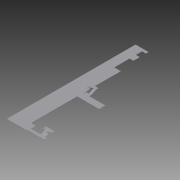
# Autodesk Inventor part: LabVIEWM0.5
Saved by Autodesk Inventor 2013 SP2 (Build 170200200, 200)
## iProperties
Created: 2014-11-17
Part Number: LabVIEWM0.5
Material: 常规
Document SubType Name: Modeling
Designer: 振胜
Density: 1 g/cm^3
Author: 振胜
Autodesk Inventor part; units mm, degrees
ref_plane "工作平面1" through (0, 0, 0) normal (0, 0, 1) x (1, 0, 0)
sketch "草图1" plane through (0, 0, 0) normal (0, 0, 1) x (1, 0, 0)
  line L0 (0, 0) -> (60, 0)
  line L1 (60, 0) -> (60, -1169.8)
  line L2 (60, -1169.8) -> (0, -1169.8)
  line L3 (0, -1169.8) -> (0, 0)
  line L4 (0, -80.6) -> (60, -80.6)
  line L5 (0, -191.9) -> (60, -191.9)
  line L6 (0, -276.5) -> (60, -276.5)
  line L7 (0, -335.9) -> (60, -335.9)
  line L8 (0, -420.6) -> (60, -420.6)
  line L9 (0, -550.6) -> (60, -550.6)
  line L10 (0, -677.8) -> (60, -677.8)
  line L11 (0, -782.9) -> (60, -782.9)
  line L12 (0, -839.5) -> (60, -839.5)
  line L13 (0, -923.6) -> (60, -923.6)
  line L14 (0, -1007.7) -> (60, -1007.7)
  line L15 (0, -1091.2) -> (60, -1091.2)
  line L16 (60, 0) -> (118.4, 0)
  line L17 (118.4, 0) -> (118.4, -23.7)
  line L18 (118.4, -23.7) -> (83.4, -23.7)
  line L19 (83.4, -23.7) -> (83.4, -79.7)
  line L20 (83.4, -79.7) -> (118.4, -79.7)
  line L21 (118.4, -79.7) -> (118.4, -137.6)
  line L22 (118.4, -137.6) -> (83.4, -137.6)
  line L23 (83.4, -137.6) -> (83.4, -276.5)
  line L24 (83.4, -276.5) -> (142.9, -276.5)
  line L25 (142.9, -276.5) -> (142.9, -379.5)
  line L26 (83.4, -276.5) -> (83.4, -379.5)
  line L27 (83.4, -379.5) -> (142.9, -379.5)
  line L28 (142.9, -379.5) -> (142.9, -463)
  line L29 (142.9, -463) -> (83.4, -463)
  line L30 (83.4, -463) -> (83.4, -379.5)
  line L31 (142.9, -463) -> (142.9, -566.2)
  line L32 (142.9, -566.2) -> (83.4, -566.2)
  line L33 (83.4, -566.2) -> (83.4, -463)
  line L34 (142.9, -566.2) -> (146.7, -566.2)
  line L35 (146.7, -566.2) -> (146.7, -616.2)
  line L36 (146.7, -616.2) -> (192.5, -616.2)
  line L37 (192.5, -616.2) -> (192.5, -673.2)
  line L38 (192.5, -616.2) -> (342.5, -616.2)
  line L39 (342.5, -616.2) -> (342.5, -673.2)
  line L40 (342.5, -673.2) -> (143.4, -673.2)
  line L41 (143.4, -673.2) -> (83.4, -673.2)
  line L42 (83.4, -673.2) -> (83.4, -1092.3)
  line L43 (83.4, -1092.3) -> (143.4, -1092.3)
  line L44 (143.4, -1092.3) -> (143.4, -673.2)
  line L45 (83.4, -754.3) -> (143.4, -754.3)
  line L46 (143.4, -837.8) -> (83.4, -837.8)
  line L47 (83.4, -893.6) -> (143.4, -893.6)
  line L48 (143.4, -978.3) -> (83.4, -978.3)
  line L49 (60, -1169.8) -> (188.1, -1169.8)
  line L50 (188.1, -1169.8) -> (188.1, -1092.3)
  line L51 (188.1, -1092.3) -> (143.4, -1092.3)
  line L52 (83.4, -1092.3) -> (83.4, -1117.3)
  line L53 (83.4, -1117.3) -> (188.1, -1117.3)
  line L54 (98.6, -1092.3) -> (98.6, -1117.3)
  line L55 (114.5, -1092.3) -> (114.5, -1117.3)
  line L56 (143.4, -1092.3) -> (143.4, -1117.3)
  line L57 (166.2, -1092.3) -> (166.2, -1117.3)
  line L58 (188.1, -1163.6) -> (336, -1163.6)
  line L59 (188.1, -1137.1) -> (336, -1137.1)
  line L60 (336, -1137.1) -> (336, -1163.6)
  dimension "d1" = 60
  dimension "d2" = 80.6
  dimension "d3" = 111.3
  dimension "d4" = 84.6
  dimension "d5" = 59.4
  dimension "d6" = 84.7
  dimension "d7" = 130
  dimension "d8" = 127.2
  dimension "d9" = 105.1
  dimension "d10" = 56.6
  dimension "d11" = 84.1
  dimension "d12" = 84.1
  dimension "d13" = 83.5
  dimension "d14" = 78.6
  dimension "d15" = 58.4
  dimension "d16" = 23.7
  dimension "d17" = 35
  dimension "d18" = 56
  dimension "d19" = 57.9
  dimension "d20" = 35
  dimension "d21" = 138.9
  dimension "d22" = 59.5
  dimension "d23" = 103
  dimension "d24" = 83.5
  dimension "d25" = 103.2
  dimension "d26" = 59.5
  dimension "d27" = 3.8
  dimension "d28" = 50
  dimension "d29" = 45.8
  dimension "d30" = 57
  dimension "d31" = 150
  dimension "d32" = 57
  dimension "d33" = 199.1
  dimension "d34" = 60
  dimension "d36" = 81.1
  dimension "d37" = 83.5
  dimension "d38" = 55.8
  dimension "d39" = 84.7
  dimension "d40" = 114
  dimension "d41" = 128.1
  dimension "d42" = 25
  dimension "d43" = 15.2
  dimension "d44" = 15.9
  dimension "d45" = 28.9
  dimension "d46" = 22.8
  dimension "d47" = 21.9
  dimension "d48" = 147.9
  dimension "d49" = 6.2
  dimension "d50" = 26.5
  constraints: 118 end point, 34 perpendicular, 19 point on line, 14 parallel, 13 horizontal, 30 other
  measures "d1" distance of L0.start L0.end
  measures "d2" distance between parallel lines of L4 L0
  measures "d3" distance between parallel lines of L5 L4
  measures "d4" distance between parallel lines of L6 L5
  measures "d5" distance between parallel lines of L7 L6
  measures "d6" distance between parallel lines of L8 L7
  measures "d7" distance between parallel lines of L9 L8
  measures "d8" distance between parallel lines of L10 L9
  measures "d9" distance between parallel lines of L11 L10
  measures "d10" distance between parallel lines of L12 L11
  measures "d11" distance between parallel lines of L13 L12
  measures "d12" distance between parallel lines of L14 L13
  measures "d13" distance between parallel lines of L15 L14
  measures "d14" distance between parallel lines of L2 L15
  measures "d15" distance of L0.end L16.end
  measures "d16" distance of L16.end L17.end
  measures "d17" distance of L17.end L18.end
  measures "d18" distance of L18.end L19.end
  measures "d19" distance of L20.end L21.end
  measures "d20" distance of L21.end L22.end
  measures "d21" distance of L22.end L23.end
  measures "d22" distance of L23.end L24.end
  measures "d23" distance of L24.end L25.end
  measures "d24" distance of L25.end L28.end
  measures "d25" distance of L28.end L31.end
  measures "d26" distance of L31.end L32.end
  measures "d27" distance of L31.end L34.end
  measures "d28" distance of L34.end L35.end
  measures "d29" distance of L35.end L36.end
  measures "d30" distance of L36.end L37.end
  measures "d31" distance of L36.end L38.end
  measures "d32" distance of L38.end L39.end
  measures "d33" distance of L39.end L40.end
  measures "d34" distance of L40.end L41.end
  measures "d36" distance between parallel lines of L45 L41
  measures "d37" distance between parallel lines of L46 L45
  measures "d38" distance between parallel lines of L47 L46
  measures "d39" distance between parallel lines of L48 L47
  measures "d40" distance between parallel lines of L43 L48
  measures "d41" distance of L2.start L49.end
  measures "d42" distance between parallel lines of L53 L51
  measures "d43" distance between parallel lines of L54 L52
  measures "d44" distance between parallel lines of L55 L54
  measures "d45" distance between parallel lines of L56 L55
  measures "d46" distance between parallel lines of L57 L56
  measures "d47" distance between parallel lines of L50 L57
  measures "d48" distance of L58.start L58.end
  measures "d49" distance between parallel lines of L49 L58
  measures "d50" distance between parallel lines of L58 L59
extrude "拉伸1" add sketch "草图1" against normal blind 1
sketch "草图2" plane through (0, 0, 0) normal (0, 0, 1) x (1, 0, 0)
  line L0 (342.5, -616.2) -> (146.7, -616.2) construction
  line L1 (342.5, -673.2) -> (342.5, -616.2) construction
  line L2 (143.4, -673.2) -> (342.5, -673.2) construction
  line L3 (146.7, -616.2) -> (146.7, -566.2) construction
  line L4 (150.3, -616.2) -> (150.3, -596.9)
  line L5 (150.3, -596.9) -> (196.1, -596.9)
  line L6 (196.1, -596.9) -> (196.1, -616.2)
  line L7 (150.3, -616.2) -> (196.1, -616.2)
  point P0 (0, 0)
  dimension "d53" = 19.3
  dimension "d54" = 45.8
  dimension "d55" = 3.6
  constraints: 8 end point, 2 perpendicular, 2 point on line, 1 collinear, 1 parallel
  measures "d53" distance of L4.start L4.end
  measures "d54" distance of L4.end L5.end
  measures "d55" distance between parallel lines of L3 L4
extrude "拉伸2" add sketch "草图2" against normal up to surface (1 mm away)
ref_plane "工作平面2" through (173.2, -616.2, 0) normal (1, 0, 0) x (0, 0, -1)
sketch "草图3" plane through (173.2, -616.2, 0) normal (1, 0, 0) x (0, 0, -1)
  line L0 (0, 19.3) -> (1, 19.3) construction
  line L1 (0.5, 19.3) -> (-20.5, 61.3)
  line L2 (0.5, 19.3) -> (0.1, 19.3)
  line L3 (0.1, 19.3) -> (-20.9, 61.3)
  line L4 (-20.9, 61.3) -> (-20.5, 61.3)
  line L5 (-20.9, 61.3) -> (-20.9, 83.8)
  line L6 (-20.9, 83.8) -> (-20.5, 83.8)
  line L7 (-20.5, 83.8) -> (-20.5, 61.3)
  point P0 (0, 616.2)
  dimension "d58" = 42
  dimension "d60" = 21
  dimension "d61" = 0.4
  dimension "d64" = 22.5
  constraints: 14 end point, 2 parallel, 1 horizontal, 1 midpoint, 1 perpendicular, 1 point on line, 1 vertical
  measures "d58" vertical distance of L1.start L1.end
  measures "d60" horizontal distance of L1.start L1.end
  measures "d61" distance of L1.start L2.end
  measures "d64" distance of L3.end L5.end
extrude "拉伸3" add sketch "草图3" along normal up to surface (22.9 mm away)
extrude "拉伸4" add sketch "草图3" against normal up to surface (22.9 mm away) contours L4 L5 L6 L7
sketch "草图5" plane through (150.3, -554.9, 20.5) normal (-1, 0, 0) x (0, 0, 1)
  line L0 (0.4, 0) -> (0, 0) construction
  line L1 (0.2, 0) -> (21.2, -42) construction
  line L2 (0, 0) -> (21, -42)
  line L3 (0.4, 0) -> (0, 0)
  line L4 (0.4, 0) -> (21.4, -42)
  line L5 (21.4, -42) -> (21.2, -42)
  line L6 (21, -42) -> (21.2, -42)
  line L7 (21.4, -42) -> (21.4, -61.3)
  line L8 (21.4, -61.3) -> (21, -61.3)
  line L9 (21, -61.3) -> (21, -42)
  point P0 (-20.5, 554.9)
  dimension "d67" = 42
  dimension "d69" = 21
  dimension "d71" = 19.3
  constraints: 18 end point, 3 equal length, 2 horizontal, 2 perpendicular, 1 midpoint, 1 vertical
  measures "d67" vertical distance of L1.start L1.end
  measures "d69" horizontal distance of L1.start L1.end
  measures "d71" distance of L4.end L7.end
extrude "拉伸5" add sketch "草图5" against normal up to surface (22.9 mm away)
ref_plane "工作平面3" through (318, -1163.6, 0) normal (1, 0, 0) x (0, 0, -1)
sketch "草图6" plane through (318, -1163.6, 0) normal (1, 0, 0) x (0, 0, -1)
  line L0 (0, 26.5) -> (1, 26.5) construction
  line L1 (0.5, 26.5) -> (-20.5, 68.5)
  line L2 (0.5, 26.5) -> (0.1, 26.5)
  line L3 (0.1, 26.5) -> (-20.9, 68.5)
  line L4 (-20.9, 68.5) -> (-20.5, 68.5)
  line L5 (-20.9, 68.5) -> (-20.9, 93.5)
  line L6 (-20.9, 93.5) -> (-20.5, 93.5)
  line L7 (-20.5, 93.5) -> (-20.5, 68.5)
  point P0 (0, 1163.6)
  dimension "d75" = 42
  dimension "d77" = 21
  dimension "d78" = 0.4
  dimension "d79" = 25
  dimension "d80" = 0.4
  constraints: 14 end point, 2 perpendicular, 1 horizontal, 1 midpoint, 1 parallel, 1 point on line
  measures "d75" vertical distance of L1.start L1.end
  measures "d77" horizontal distance of L1.start L1.end
  measures "d78" distance of L1.start L2.end
  measures "d79" distance of L3.end L5.end
  measures "d80" distance of L5.end L6.end
extrude "拉伸6" add sketch "草图6" against normal blind 40
sketch "草图7" plane through (318, -1163.6, 0) normal (1, 0, 0) x (0, 0, -1)
  line L0 (-20.9, 93.5) -> (-20.9, 68.5) construction
  line L1 (-20.5, 68.5) -> (-20.5, 93.5) construction
  line L2 (-20.5, 93.5) -> (-20.9, 93.5) construction
  line L3 (-20.9, 93.5) -> (-20.5, 93.5)
  line L4 (-20.5, 93.5) -> (-20.5, 68.5)
  line L5 (-20.5, 68.5) -> (-20.9, 68.5)
  line L6 (-20.9, 68.5) -> (-20.9, 93.5)
  line L7 (-20.5, 68.5) -> (-41.5, 26.5)
  line L8 (-20.9, 68.5) -> (-41.9, 26.5)
  line L9 (-41.9, 26.5) -> (-41.5, 26.5)
  point P0 (0, 1163.6)
  dimension "d83" = 21
  dimension "d84" = 42
  constraints: 14 end point, 3 parallel, 2 horizontal, 1 perpendicular
  measures "d83" horizontal distance of L1.start L7.end
  measures "d84" vertical distance of L1.start L7.end
extrude "拉伸7" add sketch "草图7" along normal up to surface (18 mm away)
ref_plane "工作平面4" through (298, -1163.6, 0) normal (1, 0, 0) x (0, 0, -1)
mirror "镜像1" about plane through (298, -1163.6, 0) normal (1, 0, 0) of "拉伸7"
